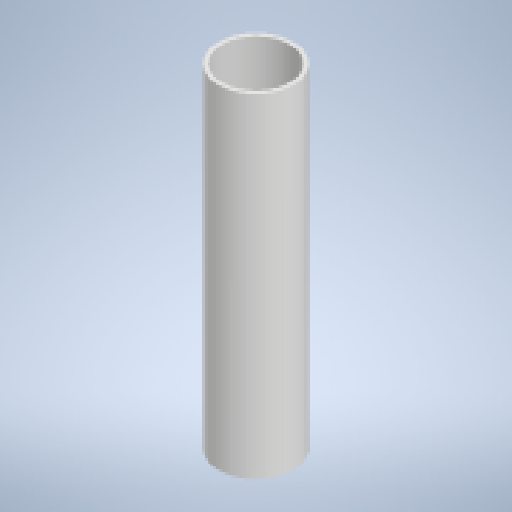
# Autodesk Inventor part: WashChamber
Saved by Autodesk Inventor 2024 (Build 280153000, 153)
## iProperties
Created: 2024-09-07
Part Number: WashChamber
Material: Generic
Document SubType Name: Modeling
Designer: Tommy Rohmann
Density: 1 g/cm^3
Appearance: Default
Link: https://www.amazon.com/gp/product/B07VD4RYXT/ref=ppx_yo_dt_b_search_asin_title?ie=UTF8&th=1
Author: Tommy Rohmann
Autodesk Inventor part; units mm, degrees
ref_plane "YZ Plane" through (0, 0, 0) normal (1, 0, 0) x (0, 1, 0)
ref_plane "XZ Plane" through (0, 0, 0) normal (0, 1, 0) x (-1, 0, 0)
ref_plane "XY Plane" through (0, 0, 0) normal (0, 0, 1) x (1, 0, 0)
sketch "Sketch1" plane through (0, 0, 0) normal (0, 1, 0) x (-1, 0, 0)
  circle A0 centre (0, 0) radius 50.8
  circle A1 centre (0, 0) radius 57.15
  dimension "WashChamberID" = 101.6
  dimension "WashChamberOD" = 114.3
  constraints: 2 centre point, 2 coincident
  measures "WashChamberID" diameter of A0
  measures "WashChamberOD" diameter of A1
extrude "Extrusion1" add sketch "Sketch1" along normal blind 508
body "Solid1"
